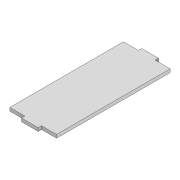
# Autodesk Inventor part: piso medio
Saved by Autodesk Inventor 2022 (Build 260153000, 153)
## iProperties
Created: 2022-06-21
Part Number: piso medio
Material: Generic
Document SubType Name: Modeling
Designer: ADMIN
Density: 1 g/cm^3
Appearance: Default
Author: ADMIN
Autodesk Inventor part; units mm, degrees
ref_plane "YZ Plane" through (0, 0, 0) normal (1, 0, 0) x (0, 1, 0)
ref_plane "XZ Plane" through (0, 0, 0) normal (0, 1, 0) x (-1, 0, 0)
ref_plane "XY Plane" through (0, 0, 0) normal (0, 0, 1) x (1, 0, 0)
sketch "Sketch1" plane through (0, 0, 0) normal (0, 1, 0) x (-1, 0, 0)
  line L0 (18.5932, 129.0225) -> (-51.4068, 129.0225)
  line L1 (-51.4068, 129.0225) -> (-51.4068, -40.9775)
  line L2 (-51.4068, -40.9775) -> (18.5932, -40.9775)
  line L3 (18.5932, -40.9775) -> (18.5932, 129.0225)
  line L4 (-3.9068, 129.0225) -> (-28.9068, 129.0225)
  line L5 (-28.9068, 129.0225) -> (-28.9068, 134.0225)
  line L6 (-28.9068, 134.0225) -> (-3.9068, 134.0225)
  line L7 (-3.9068, 134.0225) -> (-3.9068, 129.0225)
  line L8 (-3.9068, -40.9775) -> (-28.9068, -40.9775)
  line L9 (-28.9068, -40.9775) -> (-28.9068, -45.9775)
  line L10 (-28.9068, -45.9775) -> (-3.9068, -45.9775)
  line L11 (-3.9068, -45.9775) -> (-3.9068, -40.9775)
  point P0 (0, 0)
  dimension "d0" = 70
  dimension "d1" = 170
  dimension "d2" = 25
  dimension "d3" = 5
  dimension "d4" = 22.5
  dimension "d5" = 25
  dimension "d6" = 5
  constraints: 24 end point, 6 parallel, 3 horizontal, 3 perpendicular, 2 point on line
  measures "d0" distance of L2.end L1.end
  measures "d1" distance of L1.end L0.end
  measures "d2" distance of L5.end L6.end
  measures "d3" distance of L6.end L4.start
  measures "d4" distance between parallel lines of L3 L7
  measures "d5" distance of L10.end L9.end
  measures "d6" distance of L9.end L8.end
extrude "Extrusion1" add sketch "Sketch1" along normal blind 5
equation "\"d4\" = -0.5 * d2 + 0.5 * d0"
body "Solid1"
